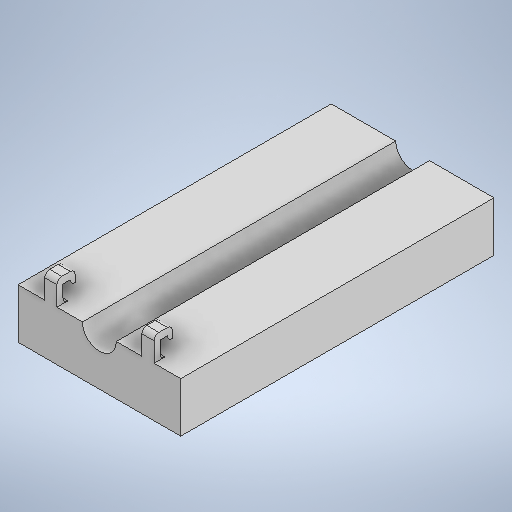
# Autodesk Inventor part: Laser_Pen_Housing
Saved by Autodesk Inventor 2025 (Build 290162000, 162)
## iProperties
Created: 2024-05-23
Part Number: Laser_Pen_Housing
Material: Generic
Document SubType Name: Modeling
Designer: mumin
Density: 1 g/cm^3
Appearance: Default
Author: mumin
Autodesk Inventor part; units mm, degrees
ref_plane "XZ Plane" through (0, 0, 0) normal (0, 1, 0) x (-1, 0, 0)
ref_plane "XY Plane" through (0, 0, 0) normal (0, 0, 1) x (1, 0, 0)
sketch "Sketch1" plane through (0, 0, 0) normal (0, 0, 1) x (1, 0, 0)
  line L0 (0, 0) -> (0, 44.0101) construction
  line L1 (33.5, 0) -> (33.5, -20.5)
  line L2 (33.5, -20.5) -> (-33.5, -20.5)
  line L3 (-33.5, -20.5) -> (-33.5, 0)
  arc A0 (-6.975, 0) -> (6.975, 0) centre (0, 0) ccw
  line L4 (-33.5, 0) -> (-6.975, 0)
  line L5 (6.975, 0) -> (33.5, 0)
  dimension "d0" = 67
  dimension "d1" = 20.5
  dimension "d2" = 6.975
  constraints: 12 end point, 3 parallel, 2 horizontal, 2 perpendicular, 2 point on circle, 1 centre point, 1 coincident, 1 vertical, 1 other
  measures "d0" distance of L1.end L2.end
  measures "d1" distance of L1.start L1.end
  measures "d2" radius of A0
extrude "Extrusion1" add sketch "Sketch1" along normal mid plane 129
ref_plane "Work Plane1" through (20, 0, 0) normal (1, 0, 0) x (0, 1, 0)
sketch "Sketch2" plane through (20, 0, 0) normal (1, 0, 0) x (0, 1, 0)
  line L0 (-6.975, 64.5) -> (0, 64.5) projected
  line L1 (0, 64.5) -> (8, 64.5)
  line L2 (7.0278, 62) -> (2, 62)
  line L3 (10, 62.5) -> (10, 59)
  line L4 (8, 57) -> (5, 57)
  arc A0 (7.0278, 58.9998) -> (5, 57) centre (7, 57) ccw
  line L5 (7.0278, 62) -> (7.0278, 58.9998)
  line L6 (0, -64.5) -> (0, 64.5) projected
  arc A1 (2, 62) -> (0, 60) centre (2, 60) ccw
  arc A2 (10, 62.5) -> (8, 64.5) centre (8, 62.5) ccw
  arc A3 (8, 57) -> (10, 59) centre (8, 59) ccw
  point P0 (0, 0)
  point P1 (10, 64.5)
  point P2 (0.0278, 62)
  point P3 (10, 57)
  dimension "d6" = 10
  dimension "d8" = 2.5
  dimension "d12" = 7
  dimension "d13" = 7.5
  dimension "d14" = 5
  dimension "d15" = 2
  dimension "d16" = 2
  dimension "d19" = 2
  constraints: 10 end point, 8 point on circle, 6 point on line, 5 tangent, 4 centre point, 2 horizontal, 2 vertical, 1 equal radius
  measures "d6" distance of L0.end point (10, 64.5)
  measures "d8" distance between parallel lines of L1 L2
  measures "d12" distance of L2.start point (0.028, 62)
  measures "d13" distance of point (10, 64.5) point (10, 57)
  measures "d14" distance of point (10, 57) L4.end
  measures "d15" distance of L4.end A0.centre
  measures "d16" radius of A1
  measures "d19" radius of A2
extrude "Extrusion2" add sketch "Sketch2" along normal mid plane 5
mirror "Mirror1" about plane through (0, 0, 0) normal (1, 0, 0) of "Extrusion2"
body "Solid1"
